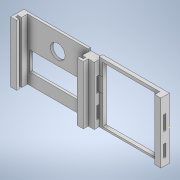
# Autodesk Inventor part: circuit clip
Saved by Autodesk Inventor 2022 (Build 260153070, 153G)
## iProperties
Created: 2022-05-13
Part Number: circuit clip
Material: Generic
Document SubType Name: Modeling
Designer: Jeanette Guo
Density: 1 g/cm^3
Appearance: Default
Author: Jeanette Guo
## iProperties of the stored document circuit clip_3DPrint.ipt
Created: 2022-05-16
Part Number: circuit clip_3DPrint
Material: Generic
Document SubType Name: Modeling
Designer: jg000189
Density: 1 g/cm^3
Appearance: Default
Author: jg000189
Autodesk Inventor part; units mm, degrees
ref_plane "YZ Plane" through (0, 0, 0) normal (1, 0, 0) x (0, 1, 0)
ref_plane "XZ Plane" through (0, 0, 0) normal (0, 1, 0) x (-1, 0, 0)
ref_plane "XY Plane" through (0, 0, 0) normal (0, 0, 1) x (1, 0, 0)
sketch "Sketch1" plane through (0, 0, 0) normal (0, 0, 1) x (1, 0, 0)
  line L0 (-60, 27.5) -> (-4, 27.5) projected
  line L1 (-60, -27.5) -> (-60, 27.5) projected
  line L2 (60, 27.5) -> (60, -27.5) projected
  line L3 (60, -27.5) -> (-60, -27.5) projected
  line L4 (10, -17) -> (50, -17) projected
  line L5 (-10, -13) -> (-10, -3) projected
  line L6 (-10, -3) -> (-20, -3) projected
  line L7 (-20, -3) -> (-20, -13) projected
  line L8 (-20, -13) -> (-10, -13) projected
  line L9 (60, -27.5) -> (-60, -27.5) projected
  line L10 (60, 27.5) -> (60, -27.5) projected
  line L11 (4, 27.5) -> (60, 27.5) projected
  arc A0 (-4, 27.5) -> (4, 27.5) centre (0, 27.5) ccw projected
  line L12 (-60, 27.5) -> (-4, 27.5) projected
  line L13 (-60, -27.5) -> (-60, 27.5) projected
  circle A1 centre (-30, 10.2208) radius 3 projected
  line L14 (50, 17) -> (10, 17) projected
  line L15 (50, -17) -> (50, 17) projected
  line L16 (10, -17) -> (50, -17) projected
  line L17 (10, 17) -> (10, -17) projected
  line L18 (-40, -3) -> (-50, -3) projected
  line L19 (-40, -13) -> (-40, -3) projected
  line L20 (-50, -13) -> (-40, -13) projected
  line L21 (-50, -3) -> (-50, -13) projected
  line L22 (-25, -3) -> (-35, -3) projected
  line L23 (-25, -13) -> (-25, -3) projected
  line L24 (-35, -13) -> (-25, -13) projected
  line L25 (-35, -3) -> (-35, -13) projected
  line L26 (-10, -3) -> (-20, -3) projected
  line L27 (-10, -13) -> (-10, -3) projected
  line L28 (-20, -13) -> (-10, -13) projected
  line L29 (-20, -3) -> (-20, -13) projected
  line L30 (-35, -13) -> (-25, -13) projected
  line L31 (-35, -3) -> (-35, -13) projected
  circle A2 centre (-30, 10.2208) radius 3 projected
  line L32 (-60, 27.5) -> (60, 27.5)
  line L33 (60, 27.5) -> (60, -27.5)
  line L34 (60, -27.5) -> (-60, -27.5)
  line L35 (-60, -27.5) -> (-60, 27.5)
  line L36 (10, 17) -> (50, 17)
  line L37 (50, 17) -> (50, -17)
  line L38 (50, -17) -> (10, -17)
  line L39 (10, -17) -> (10, 17)
  line L40 (-50, -3) -> (-40, -3)
  line L41 (-40, -3) -> (-40, -13)
  line L42 (-40, -13) -> (-50, -13)
  line L43 (-50, -13) -> (-50, -3)
  line L44 (-35, -3) -> (-25, -3)
  line L45 (-25, -3) -> (-25, -13)
  line L46 (-25, -13) -> (-35, -13)
  line L47 (-35, -13) -> (-35, -3)
  line L48 (-20, -3) -> (-10, -3)
  line L49 (-10, -3) -> (-10, -13)
  line L50 (-10, -13) -> (-20, -13)
  line L51 (-20, -13) -> (-20, -3)
  circle A3 centre (-30, 10.2208) radius 3
  arc A4 (-4, 27.5) -> (4, 27.5) centre (0, 27.5) ccw
  point P0 (0, 0)
  dimension "d0" = 6
  constraints: 40 end point, 10 parallel, 5 horizontal, 5 perpendicular, 2 centre point, 2 point on circle, 1 coincident, 1 concentric
  measures "d0" diameter of A3
extrude "Extrusion1" add sketch "Sketch1" along normal blind 3 contours L0 A0 L11 L2 L3 L1
sketch "Sketch2" plane through (0, 0, 3) normal (0, 0, 1) x (1, 0, 0)
  line L0 (10, 17) -> (50, 17) projected
  line L1 (8, 22) -> (51, 22)
  line L2 (51, 22) -> (51, -24)
  line L3 (51, -24) -> (8, -24)
  line L4 (8, -24) -> (8, 22)
  line L5 (10, -17) -> (10, 17) projected
  line L6 (50, -17) -> (10, -17) projected
  line L7 (50, 17) -> (50, -17) projected
  circle A0 centre (-30, 10.2208) radius 3 projected
  circle A1 centre (-30, 10.2208) radius 6
  line L8 (-53, 0) -> (-7, 0)
  line L9 (-7, 0) -> (-7, -16)
  line L10 (-7, -16) -> (-53, -16)
  line L11 (-53, -16) -> (-53, 0)
  line L12 (-50, -13) -> (-50, -3) projected
  line L13 (-40, -13) -> (-50, -13) projected
  line L14 (-25, -13) -> (-35, -13) projected
  line L15 (-10, -3) -> (-10, -13) projected
  line L16 (-10, -13) -> (-20, -13) projected
  line L17 (-35, -3) -> (-25, -3) projected
  point P0 (0, 0)
  dimension "d4" = 5
  dimension "d5" = 2
  dimension "d6" = 7
  dimension "d7" = 1
  dimension "d10" = 12
  dimension "d11" = 3
  dimension "d12" = 3
  dimension "d13" = 3
  dimension "d14" = 3
  constraints: 16 end point, 4 parallel, 2 horizontal, 2 perpendicular, 1 centre point, 1 coincident
  measures "d4" distance between parallel lines of L1 L0
  measures "d5" distance between parallel lines of L4 L5
  measures "d6" distance between parallel lines of L3 L6
  measures "d7" distance between parallel lines of L7 L2
  measures "d10" diameter of A1
  measures "d11" distance between parallel lines of L11 L12
  measures "d12" distance between parallel lines of L9 L15
  measures "d13" distance between parallel lines of L10 L14
  measures "d14" distance between parallel lines of L8 L17
extrude "Extrusion2" cut sketch "Sketch2" against normal blind 3
sketch "Sketch6" plane through (0, 0, 3) normal (0, 0, 1) x (1, 0, 0)
  line L0 (-60, 27.5) -> (-60, -27.5) projected
  line L1 (-60, -27.5) -> (60, -27.5) projected
  line L2 (-60, 27.5) -> (-55, 27.5)
  line L3 (-55, 27.5) -> (-55, -27.5)
  line L4 (-55, -27.5) -> (-60, -27.5)
  line L5 (-60, -27.5) -> (-60, 27.5)
  line L6 (-4, 27.5) -> (-60, 27.5) projected
  line L7 (0, -27.5) -> (-5, -27.5)
  line L8 (-5, -27.5) -> (-5, 27.5)
  line L9 (-5, 27.5) -> (0, 27.5)
  line L10 (0, 27.5) -> (0, -27.5)
  arc A0 (-4, 27.5) -> (4, 27.5) centre (0, 27.5) ccw projected
  point P0 (0, 0)
  point P1 (0, -27.5)
  point P2 (-5, -27.5)
  point P3 (0, 23.5)
  dimension "d23" = 5
  dimension "d24" = 5
  constraints: 16 end point, 4 parallel, 3 point on line, 2 horizontal, 2 perpendicular, 1 point on circle, 1 vertical alignment
  measures "d23" distance of L3.end L4.end
  measures "d24" distance of L8.end L9.end
extrude "Extrusion5" add sketch "Sketch6" along normal blind 8 contours L2 L3 L1 L0 | L6 A0 L10 L1 L8 | L9 L10 A0
sketch "Sketch7" plane through (-60, 27.5, 0) normal (0, 1, 0) x (1, 0, 0)
  line L0 (5, -3) -> (5, -11) construction
  line L1 (5, -3) -> (5, -7) construction
  line L2 (5, -7) -> (2, -7)
  line L3 (2, -7) -> (2, -9)
  line L4 (2, -9) -> (5, -9)
  line L5 (55, -3) -> (5, -3) projected
  line L6 (30, -3) -> (30, -9) construction
  line L7 (55, -3) -> (55, -11) construction
  line L8 (55, -3) -> (55, -7) construction
  line L9 (55, -7) -> (58, -7)
  line L10 (58, -7) -> (58, -9)
  line L11 (58, -9) -> (55, -9)
  line L12 (5, -7) -> (5, -9)
  line L13 (55, -7) -> (55, -9)
  point P0 (60, 0)
  dimension "d27" = 4
  dimension "d28" = 3
  dimension "d29" = 2
  constraints: 24 end point, 5 symmetric about line, 3 midpoint, 2 collinear, 2 perpendicular, 2 point on line, 1 horizontal, 1 vertical
  measures "d27" distance of L0.start L1.end
  measures "d28" distance of L1.end L2.end
  measures "d29" distance of L2.end L3.end
extrude "Extrusion6" cut sketch "Sketch7" against normal through all
sketch "Sketch10" plane through (0, 0, 3) normal (0, 0, 1) x (1, 0, 0)
  line L0 (-55, -27.5) -> (-55, 27.5) projected
  line L1 (-5, 27.5) -> (-5, -27.5) projected
  line L2 (-55, 27.5) -> (-5, 27.5)
  line L3 (-5, 27.5) -> (-5, -27.5)
  line L4 (-5, -27.5) -> (-55, -27.5)
  line L5 (-55, -27.5) -> (-55, 27.5)
  point P0 (0, 0)
  constraints: 8 end point, 2 parallel, 1 horizontal, 1 perpendicular
extrude "Extrusion9" cut sketch "Sketch10" against normal blind 1
sketch "Sketch11" plane through (0, 0, 3) normal (0, 0, 1) x (1, 0, 0)
  line L0 (0, -27.5) -> (0, 27.5) projected
  line L1 (-60, -27.5) -> (60, -27.5) projected
  line L2 (0, 27.5) -> (5, 27.5)
  line L3 (5, 27.5) -> (5, -27.5)
  line L4 (5, -27.5) -> (0, -27.5)
  line L5 (0, -27.5) -> (0, 27.5)
  line L6 (60, -27.5) -> (60, 27.5) projected
  line L7 (60, 27.5) -> (55, 27.5)
  line L8 (55, 27.5) -> (55, -27.5)
  line L9 (55, -27.5) -> (60, -27.5)
  line L10 (60, -27.5) -> (60, 27.5)
  point P0 (0, 0)
  dimension "d43" = 5
  dimension "d44" = 5
  constraints: 16 end point, 4 parallel, 2 horizontal, 2 perpendicular, 2 point on line
  measures "d43" distance of L3.end L4.end
  measures "d44" distance of L9.end L8.end
extrude "Extrusion10" add sketch "Sketch11" along normal blind 4
sketch "Sketch14" plane through (60, -27.5, 0) normal (1, 0, 0) x (0, 0, -1)
  point P0 (0, 27.5)
sketch "Sketch15" plane through (60, -27.5, 0) normal (1, 0, 0) x (0, 0, -1)
  line L0 (-2, 55) -> (-2, 0) projected
  line L1 (-7, 0) -> (-2, 0) projected
  line L2 (-3.0003, 0.0005) -> (-3.0003, 18)
  line L3 (-2, 0) -> (-2, 55) projected
  line L4 (-3.0003, 18) -> (-5.0003, 18)
  line L5 (-5.0003, 18) -> (-5.0003, 8)
  line L6 (-5.0003, 8) -> (-3.0003, 8)
  line L7 (-2.9987, 54.9727) -> (-2.9987, 27)
  line L8 (-2.9987, 27) -> (-5.0003, 27)
  line L9 (-5.0003, 27) -> (-5.0003, 39)
  line L10 (-5.0003, 39) -> (-2.9987, 39)
  line L11 (-3, 0) -> (-3, 55) projected
  line L12 (0, 55) -> (-7, 55) projected
  point P0 (0, 27.5)
  point P1 (-2, 39)
  point P2 (-2, 8)
  point P3 (-2, 18)
  dimension "d65" = 2
  dimension "d66" = 10
  dimension "d68" = 12
  dimension "d71" = 28
  dimension "d72" = 18
  constraints: 16 end point, 5 perpendicular, 4 point on line
  measures "d65" distance of L2.end L4.end
  measures "d66" distance of L4.end L5.end
  measures "d68" distance of L8.end L9.end
  measures "d71" distance between parallel lines of L12 L8
  measures "d72" distance between parallel lines of L1 L4
extrude "Extrusion13" cut sketch "Sketch15" against normal up to surface (60 mm away) contours L6 L5 L4 L2 | L7 L8 L9 L10
sketch "Sketch16" plane through (0, 0, 11) normal (0, 0, 1) x (1, 0, 0)
  line L0 (-60, 27.5) -> (-60, -27.5) projected
  line L1 (60, -27.5) -> (60, 27.5) projected
  line L2 (-60, 27.5) -> (60, 27.5)
  line L3 (60, 27.5) -> (60, 24.5)
  line L4 (60, 24.5) -> (-60, 24.5)
  line L5 (-60, 24.5) -> (-60, 27.5)
  line L6 (-60, -27.5) -> (60, -27.5) projected
  line L7 (-60, -27.5) -> (60, -27.5)
  line L8 (60, -27.5) -> (60, -25.5)
  line L9 (60, -25.5) -> (-60, -25.5)
  line L10 (-60, -25.5) -> (-60, -27.5)
  line L11 (-55, 27.5) -> (-5, 27.5) projected
  line L12 (5, 27.5) -> (5, 11.5) projected
  line L13 (-5, 27.5) -> (5, 27.5)
  line L14 (5, 27.5) -> (5, 24.5)
  line L15 (5, 24.5) -> (-5, 24.5)
  line L16 (-5, 24.5) -> (-5, 27.5)
  line L17 (-5, 24.5) -> (5, 24.5)
  line L18 (5, 24.5) -> (5, 22.5)
  line L19 (5, 22.5) -> (-5, 22.5)
  line L20 (-5, 22.5) -> (-5, 24.5)
  point P0 (0, 0)
  point P1 (-60, -25.5)
  dimension "d74" = 3
  dimension "d77" = 2
  dimension "d78" = 2
  constraints: 32 end point, 8 parallel, 5 point on line, 4 horizontal, 4 perpendicular
  measures "d74" distance of L2.end L3.end
  measures "d77" distance of L8.end L7.end
  measures "d78" distance of L17.end L18.end
extrude "Extrusion14" cut sketch "Sketch16" against normal through all contours L2 L16 L4 L0 | L9 L1 L6 L0 | L16 L2 L12 L4 | L4 L12 L19 L20 | L12 L2 L1 L4
body "Solid1"
